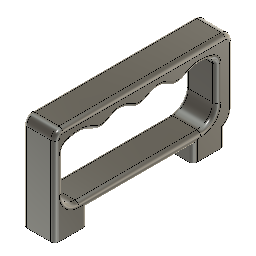
main (Autodesk Fusion 360 archive; units mm, degrees)
design "main_handle"
Autodesk Fusion 360 part; units mm, degrees
sketch "Skizze1" plane through (0, 0, 0) normal (1, 0, 0) x (0, 1, 0)
  line L0 (0, 0) -> (0, 60)
  line L1 (0, 60) -> (111.25, 60)
  line L2 (111.25, 60) -> (111.25, 10)
  line L3 (111.25, 10) -> (106.25, 10)
  line L4 (106.25, 10) -> (106.25, 0)
  line L5 (106.25, 0) -> (86.25, 0)
  line L6 (86.25, 0) -> (86.25, 10)
  line L7 (86.25, 10) -> (20, 10)
  line L8 (20, 10) -> (20, 0)
  line L9 (20, 0) -> (0, 0)
  dimension "d1" = 20
  dimension "d2" = 20
  dimension "d3" = 86.25
  dimension "d4" = 5
  dimension "d5" = 60
  dimension "d6" = 10
  dimension "d7" = 10
  constraint coincident L0.start L9.end
  constraint vertical L0
  constraint perpendicular L0 L1
  constraint perpendicular L1 L2
  constraint perpendicular L2 L3
  constraint perpendicular L3 L4
  constraint perpendicular L4 L5
  constraint perpendicular L3 L6
  constraint perpendicular L6 L7
  constraint perpendicular L3 L8
  constraint perpendicular L0 L9
  constraint collinear L5 L9
  measures "d1" distance of L8.end L0.start
  measures "d2" distance of L4.end L5.end
  measures "d3" distance of L0 L6
  measures "d4" distance of L2.end L3.end
  measures "d5" distance of L0.start L0.end
  measures "d6" distance of L7.end L8.end
  measures "d7" distance of L3.end L4.end
extrude "Extrusion1" add sketch "Skizze1" along normal mid plane 20
sketch "Skizze2" plane through (10, 0, 0) normal (1, 0, 0) x (0, 1, 0)
  line L0 (20, 0) -> (20, 10)
  line L1 (20, 10) -> (86.25, 10)
  line L2 (86.25, 10) -> (86.25, 0)
  line L3 (86.25, 0) -> (106.25, 0)
  line L4 (106.25, 0) -> (106.25, 10)
  line L5 (106.25, 10) -> (111.25, 10)
  line L6 (111.25, 10) -> (111.25, 60)
  line L7 (111.25, 60) -> (0, 60)
  line L8 (0, 60) -> (0, 0)
  line L9 (0, 0) -> (20, 0)
  spline S0 degree 5 poles (5, 50) (5.4629, 50.1553) (6.3735, 50.4513) (7.694, 50.8519) (9.3638, 51.2991) (11.3005, 51.7132) (13.0897, 51.9831) (14.7376, 52.1102) (16.2549, 52.0972) (17.6578, 51.9482) (18.9696, 51.669) (20.2192, 51.2688) (21.4368, 50.7637) (22.6495, 50.1803) (23.8773, 49.5586) (25.128, 48.9571) (26.3991, 48.445) (27.6823, 48.0889) (28.9673, 47.9419) (30.2456, 48.0313) (31.5144, 48.3467) (32.7751, 48.8486) (34.0317, 49.4766) (35.2885, 50.1586) (36.5487, 50.8196) (37.8129, 51.3893) (39.0803, 51.8072) (40.349, 52.0283) (41.6173, 52.0271) (42.8839, 51.8047) (44.1488, 51.3883) (45.4125, 50.8244) (46.6756, 50.1733) (47.9391, 49.5031) (49.2032, 48.8845) (50.4682, 48.3839) (51.7339, 48.0572) (53, 47.9433) (54.2661, 48.0572) (55.5318, 48.3839) (56.7968, 48.8845) (58.0609, 49.5031) (59.3244, 50.1733) (60.5875, 50.8244) (61.8512, 51.3883) (63.1161, 51.8047) (64.3827, 52.0271) (65.651, 52.0283) (66.9197, 51.8072) (68.1871, 51.3893) (69.4513, 50.8196) (70.7115, 50.1586) (71.9683, 49.4766) (73.2249, 48.8486) (74.4856, 48.3467) (75.7544, 48.0313) (77.0327, 47.9419) (78.3177, 48.0889) (79.6009, 48.445) (80.872, 48.9571) (82.1227, 49.5586) (83.3505, 50.1803) (84.5632, 50.7637) (85.7808, 51.2688) (87.0304, 51.669) (88.3422, 51.9482) (89.7451, 52.0972) (91.2624, 52.1102) (92.9103, 51.9831) (94.6995, 51.7132) (96.6362, 51.2991) (98.306, 50.8519) (99.6265, 50.4513) (100.5371, 50.1553) (101, 50) knots 0 0 0 0 0 0 0.01428571 0.02857143 0.04285714 0.05714286 0.07142857 0.08571429 0.1 0.11428571 0.12857143 0.14285714 0.15714286 0.17142857 0.18571429 0.2 0.21428571 0.22857143 0.24285714 0.25714286 0.27142857 0.28571429 0.3 0.31428571 0.32857143 0.34285714 0.35714286 0.37142857 0.38571429 0.4 0.41428571 0.42857143 0.44285714 0.45714286 0.47142857 0.48571429 0.5 0.51428571 0.52857143 0.54285714 0.55714286 0.57142857 0.58571429 0.6 0.61428571 0.62857143 0.64285714 0.65714286 0.67142857 0.68571429 0.7 0.71428571 0.72857143 0.74285714 0.75714286 0.77142857 0.78571429 0.8 0.81428571 0.82857143 0.84285714 0.85714286 0.87142857 0.88571429 0.9 0.91428571 0.92857143 0.94285714 0.95714286 0.97142857 0.98571429 1 1 1 1 1 1
  line L10 (5, 50) -> (101, 50)
  line L11 (5, 50) -> (5, 15)
  line L12 (5, 15) -> (101, 15)
  line L13 (101, 15) -> (101, 50)
  point P0 (17, 52)
  point P1 (23, 50)
  point P2 (29, 48)
  point P3 (35, 50)
  point P4 (41, 52)
  point P5 (47, 50)
  point P6 (53, 48)
  point P7 (59, 50)
  point P8 (65, 52)
  point P9 (71, 50)
  point P10 (77, 48)
  point P11 (83, 50)
  point P12 (89, 52)
  dimension "d10" = 5
  dimension "d11" = 12
  dimension "d12" = 6
  dimension "d13" = 6
  dimension "d14" = 6
  dimension "d15" = 6
  dimension "d16" = 6
  dimension "d17" = 6
  dimension "d18" = 6
  dimension "d19" = 6
  dimension "d20" = 6
  dimension "d21" = 6
  dimension "d22" = 6
  dimension "d24" = 10
  dimension "d25" = 10
  dimension "d26" = 6
  dimension "d27" = 12
  dimension "d28" = 2
  dimension "d29" = 2
  dimension "d30" = 2
  dimension "d31" = 2
  dimension "d32" = 2
  dimension "d33" = 2
  dimension "d34" = 2
  dimension "d35" = 35
  constraint coincident P1 L10
  constraint coincident P3 L10
  constraint coincident P5 L10
  constraint coincident P7 L10
  constraint coincident P9 L10
  constraint coincident P11 L10
  constraint perpendicular L10 L11
  constraint perpendicular L11 L12
  constraint perpendicular L10 L13
  measures "d10" distance of L8 S0.start
  measures "d11" distance of S0.start P0
  measures "d12" horizontal distance of P0 P1
  measures "d13" horizontal distance of P1 P2
  measures "d14" horizontal distance of P2 P3
  measures "d15" horizontal distance of P3 P4
  measures "d16" horizontal distance of P4 P5
  measures "d17" horizontal distance of P5 P6
  measures "d18" horizontal distance of P6 P7
  measures "d19" horizontal distance of P7 P8
  measures "d20" horizontal distance of P8 P9
  measures "d21" horizontal distance of P9 P10
  measures "d22" horizontal distance of P10 P11
  measures "d24" distance of L7 S0.end
  measures "d25" distance of L7 S0.start
  measures "d26" horizontal distance of P11 P12
  measures "d27" distance of S0.end P12
  measures "d28" distance of L10 P12
  measures "d29" distance of P10 L10
  measures "d30" distance of P8 L10
  measures "d31" distance of P6 L10
  measures "d32" distance of P4 L10
  measures "d33" distance of P2 L10
  measures "d34" distance of P0 L10
  measures "d35" distance of S0.start L11.end
extrude "Extrusion2" cut sketch "Skizze2" against normal through all contours S0 L10 | S0 L10 L11 L12 L13 | S0 L10 | S0 L10 | S0 L10 picked at (13.1167, 50.5643) picked at (39.3753, 50.6892) picked at (93.7853, 50.364) picked at (66.4503, 50.2815)
fillet "Abrundung11" radius 10 3 edges at (0, 101, 15) (0, 111.25, 10) (0, 5, 15)
fillet "Abrundung12" radius 5 2 edges at (0, 111.25, 60) (0, 0, 60)
fillet "Abrundung13" radius 5 2 edges at (0, 101, 50) (0, 5, 50)
fillet "Abrundung14" radius 2.5 28 edges at (-10, 0, 27.5) (-10, 1.4645, 58.5355) (-10, 55.625, 60) (-10, 109.7855, 58.5355) (-10, 111.25, 36.8301) (-10, 109.9103, 13.6603) (-10, 6.0478, 49.3407) (-10, 53, 48) (-10, 99.9489, 49.3449) (-10, 101, 35.639) (-10, 98.0711, 17.9289) (-10, 53, 15) (-10, 7.9289, 17.9289) (-10, 5, 35.639) (10, 7.9289, 17.9289) (10, 53, 15) (10, 98.0711, 17.9289) (10, 101, 35.639) (10, 99.9522, 49.3407) (10, 53, 48) (10, 6.0511, 49.3449) (10, 5, 35.639) (10, 109.9103, 13.6603) (10, 111.25, 36.8301) (10, 109.7855, 58.5355) (10, 55.625, 60) (10, 1.4645, 58.5355) (10, 0, 27.5)
fillet "Abrundung15" radius 2.5 2 edges at (-10, 53.125, 10) (10, 53.125, 10)
fillet "Abrundung16" radius 2.5 6 edges at (-10, 86.25, 6.25) (10, 86.25, 6.25) (10, 106.25, 6.535) (-10, 106.25, 6.535) (-10, 20, 6.25) (10, 20, 6.25)
sketch "Skizze3" plane through (0, 0, 0) normal (0, 0, -1) x (1, 0, 0)
  arc A0 (-10, -103.75) -> (-7.5, -106.25) centre (-7.5, -103.75) ccw
  line L0 (-7.5, -106.25) -> (7.5, -106.25)
  arc A1 (7.5, -106.25) -> (10, -103.75) centre (7.5, -103.75) ccw
  line L1 (10, -103.75) -> (10, -88.75)
  arc A2 (10, -88.75) -> (7.5, -86.25) centre (7.5, -88.75) ccw
  line L2 (7.5, -86.25) -> (-7.5, -86.25)
  arc A3 (-7.5, -86.25) -> (-10, -88.75) centre (-7.5, -88.75) ccw
  line L3 (-10, -88.75) -> (-10, -103.75)
  line L4 (0, -1.75) -> (0, -22.5)
  point P0 (0, -96.25)
  point P1 (0, -10)
  dimension "d69" = 86.25
  dimension "d70" = 10
  constraint coincident P1 L4
  constraint coincident P0 L4
  measures "d69" distance of P0 P1
  measures "d70" distance of L0 P0
hole "Bohrung1" at (0, 96.25, 0) at (0, 10, 0) direction (0, 0, 1) diameter 3.2 depth 14 tip angle 180
ref_plane "Arbeitsebene2" through (0, 96.25, 5) normal (0, 0, -1) x (0, 1, 0)
sketch "Skizze12" plane through (0, 96.25, 5) normal (0, 0, -1) x (1, 0, 0)
  line L0 (2.9, 89.85) -> (-2.9, 89.85)
  line L1 (-2.9, 89.85) -> (-2.9, -3.6)
  line L2 (-2.9, -3.6) -> (2.9, -3.6)
  line L3 (2.9, -3.6) -> (2.9, 89.85)
  point P0 (-1.6, 86.25)
  dimension "d119" = 5.8
  dimension "d120" = 3.6
  dimension "d121" = 2.9
  dimension "d122" = 3.6
  constraint horizontal L0
  constraint vertical L1
  constraint horizontal L2
  constraint vertical L3
  measures "d119" distance of L1.end L2.end
  measures "d120" distance of origin L2
  measures "d121" distance of origin L3
  measures "d122" vertical distance of L0.end P0
extrude "Extrusion10" cut sketch "Skizze12" against normal blind 3
sketch "Skizze13" plane through (0, 0, 0) normal (1, 0, 0) x (0, 1, 0)
  line L0 (111.25, 18.6603) -> (111.25, 55)
  line L1 (88.75, 0) -> (103.75, 0)
  line L2 (111.25, 50) -> (106.75, 50)
  line L3 (106.75, 50) -> (106.75, 45)
  line L4 (106.75, 45) -> (104.75, 45)
  line L5 (104.75, 45) -> (104.75, 19.017)
  line L6 (104.75, 19.017) -> (102.25, 15.4466)
  line L7 (102.25, 15.4466) -> (102.25, 0)
  line L8 (105.25, 0) -> (105.25, 14.5007)
  line L9 (105.25, 14.5007) -> (107, 17)
  line L10 (107, 17) -> (107, 42.5)
  line L11 (107, 42.5) -> (108.25, 42.5)
  line L12 (108.25, 42.5) -> (108.25, 43.5)
  line L13 (108.25, 43.5) -> (111.25, 43.5)
  line L14 (111.25, 43.5) -> (111.25, 50)
  line L15 (106.25, 60) -> (5, 60)
  line L16 (102.25, 0) -> (105.25, 0)
  dimension "d128" = 4.5
  dimension "d129" = 2
  dimension "d130" = 3
  dimension "d131" = 2.25
  dimension "d132" = 2.5
  dimension "d133" = 5
  dimension "d134" = 6.5
  dimension "d135" = 10
  dimension "d137" = 145
  dimension "d138" = 2.5
  dimension "d139" = 3
  dimension "d140" = 3
  dimension "d141" = 28
  constraint coincident L0 L2.start
  constraint perpendicular L0 L2
  constraint perpendicular L2 L3
  constraint perpendicular L3 L4
  constraint perpendicular L4 L5
  constraint coincident L1 L7.end
  constraint perpendicular L1 L7
  constraint coincident L1 L8.start
  constraint perpendicular L1 L8
  constraint parallel L6 L9
  constraint perpendicular L1 L10
  constraint perpendicular L7 L11
  constraint perpendicular L11 L12
  constraint coincident L0 L13.end
  constraint perpendicular L0 L13
  measures "d128" distance of L2.start L2.end
  measures "d129" distance of L3.end L4.end
  measures "d130" distance of L12.end L13.end
  measures "d131" distance of L5 L10
  measures "d132" distance of L4 L11
  measures "d133" distance of L2.end L3.end
  measures "d134" distance of L2.start L13.end
  measures "d135" distance of L2 L15
  measures "d137" angle of L5 L6
  measures "d138" horizontal distance of L5.end L6.end
  measures "d139" distance of L7 L8
  measures "d140" distance of L6 L9
  measures "d141" vertical distance of L4.end L9.end
extrude "Extrusion11" cut sketch "Skizze13" along normal mid plane 6.5
equation "d11 = fingerdist * 2"
equation "d12 = fingerdist"
equation "d13 = fingerdist"
equation "d14 = fingerdist"
equation "d15 = fingerdist"
equation "d16 = fingerdist"
equation "d17 = fingerdist"
equation "d18 = fingerdist"
equation "d19 = fingerdist"
equation "d20 = fingerdist"
equation "d21 = fingerdist"
equation "d22 = fingerdist"
equation "d26 = fingerdist"
equation "d27 = fingerdist * 2"
equation "fingerdist = 6 mm"

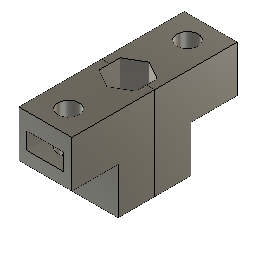
design "module_stand"
Autodesk Fusion 360 part; units mm, degrees
sketch "Skizze1" plane through (0, 0, 0) normal (1, 0, 0) x (0, 1, 0)
  line L0 (0, 0) -> (0, 14)
  line L1 (0, 14) -> (12.5, 14)
  line L2 (12.5, 14) -> (12.5, 7)
  line L3 (12.5, 7) -> (5.5, 7)
  line L4 (5.5, 7) -> (5.5, 0)
  line L5 (5.5, 0) -> (0, 0)
  dimension "d1" = 5.5
  dimension "d2" = 7
  dimension "d3" = 14
  dimension "d4" = 12.5
  constraint coincident L0.start L5.end
  constraint vertical L0
  constraint perpendicular L0 L1
  constraint perpendicular L1 L2
  constraint perpendicular L2 L3
  constraint perpendicular L1 L4
  constraint perpendicular L4 L5
  measures "d1" distance of L0.start L4.end
  measures "d2" distance of L3.end L4.end
  measures "d3" distance of L0.start L0.end
  measures "d4" distance of L0.end L1.end
extrude "Extrusion1" add sketch "Skizze1" along normal blind 8 makes body 1
sketch "Skizze2" plane through (0, 0, 14) normal (0, 0, 1) x (-1, 0, 0)
  line L0 (0, -12.5) -> (0, 0)
  line L1 (0, 0) -> (-8, 0)
  line L2 (-8, 0) -> (-8, -12.5)
  line L3 (-8, -12.5) -> (0, -12.5)
  point P0 (-4, 0)
  point P1 (-4, -9)
  dimension "d7" = 4
  dimension "d8" = 4
  dimension "d10" = 3.5
  constraint coincident L1 P0
  measures "d7" distance of L2 P1
  measures "d8" distance of L2 P0
  measures "d10" distance of L3 P1
hole "Bohrung1" at (4, 0, 14) at (4, 9, 14) direction (0, 0, -1) diameter 3.2 end through all bodies 1
sketch "Skizze3" plane through (0, 0, 14) normal (0, 0, 1) x (-1, 0, 0)
  arc A0 (-5.6, 0) -> (-2.4, 0) centre (-4, 0) ccw
  line L0 (-5.6, 0) -> (-8, 0)
  line L1 (-8, 0) -> (-8, -12.5)
  line L2 (-8, -12.5) -> (0, -12.5)
  line L3 (0, -12.5) -> (0, 0)
  line L4 (0, 0) -> (-2.4, 0)
  circle A1 centre (-4, -9) radius 1.6
  line L5 (-1.2, 1.6166) -> (-4, 3.2332)
  line L6 (-4, 3.2332) -> (-6.8, 1.6166)
  line L7 (-6.8, 1.6166) -> (-6.8, -1.6166)
  line L8 (-6.8, -1.6166) -> (-4, -3.2332)
  line L9 (-4, -3.2332) -> (-1.2, -1.6166)
  line L10 (-1.2, -1.6166) -> (-1.2, 1.6166)
  point P0 (-4, 0)
  dimension "d14" = 5.6
  constraint coincident P0 A0.centre
  constraint parallel L1 L7
  measures "d14" distance of L7 L10
extrude "Extrusion2" cut sketch "Skizze3" against normal blind 7 contours A0 L0 L4 L7 L8 L9 L10 bodies 1
sketch "Skizze5" plane through (0, 12.5, 0) normal (0, 1, 0) x (-1, 0, 0)
  line L0 (0, 7) -> (0, 14)
  line L1 (0, 14) -> (-8, 14)
  line L2 (-8, 14) -> (-8, 7)
  line L3 (-8, 7) -> (0, 7)
  line L4 (-6.8, 11.5) -> (-1.2, 11.5)
  line L5 (-1.2, 11.5) -> (-1.2, 8.9)
  line L6 (-1.2, 8.9) -> (-6.8, 8.9)
  line L7 (-6.8, 8.9) -> (-6.8, 11.5)
  dimension "d22" = 5.6
  dimension "d23" = 2.6
  dimension "d24" = 2.5
  dimension "d25" = 1.2
  dimension "d26" = 8
  constraint horizontal L4
  constraint vertical L5
  constraint horizontal L6
  constraint vertical L7
  measures "d22" distance of L5.end L6.end
  measures "d23" distance of L4.end L5.end
  measures "d24" distance of L1 L4
  measures "d25" distance of L0 L5
  measures "d26" distance of L0.end L1.end
extrude "Extrusion4" cut sketch "Skizze5" against normal blind 6.7 contours L4 L5 L6 L7 bodies 1
mirror "Spiegeln1" about plane through (0, 0, 0) normal (0, -1, 0) of "Extrusion1", "Bohrung1", "Extrusion2", "Extrusion4" makes body 2
equation "d1 = ( 11 / 2 ) * 1 mm"
equation "d4 = ( 25 / 2 ) * 1 mm"
equation "d25 = ( 8.00 mm - d22 ) / 2"

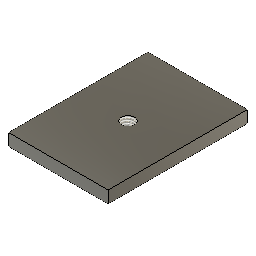
design "module_plate"
Autodesk Fusion 360 part; units mm, degrees
sketch "Skizze1" plane through (0, 0, 0) normal (0, 0, 1) x (1, 0, 0)
  line L0 (-12.5, -17.5) -> (12.5, -17.5)
  line L1 (12.5, -17.5) -> (12.5, 17.5)
  line L2 (12.5, 17.5) -> (-12.5, 17.5)
  line L3 (-12.5, 17.5) -> (-12.5, -17.5)
  dimension "d1" = 25
  dimension "d2" = 35
  dimension "d3" = 17.5
  dimension "d4" = 12.5
  constraint horizontal L0
  constraint vertical L1
  constraint horizontal L2
  constraint vertical L3
  measures "d1" distance of L0.start L0.end
  measures "d2" distance of L0.end L1.end
  measures "d3" distance of origin L2
  measures "d4" distance of origin L3
extrude "Extrusion1" add sketch "Skizze1" along normal blind 3
sketch "Skizze2" plane through (0, 0, 3) normal (0, 0, 1) x (-1, 0, 0)
  line L0 (12.5, -17.5) -> (12.5, 17.5)
  line L1 (12.5, 17.5) -> (-12.5, 17.5)
  line L2 (-12.5, 17.5) -> (-12.5, -17.5)
  line L3 (-12.5, -17.5) -> (12.5, -17.5)
hole "Bohrung1" at (0, 0, 3) direction (0, 0, -1) diameter 3.332 end through all
thread "Gewinde1" "ISO Metric profile 4.0 M4x0.7 6H"
equation "d3 = ( 35 / 2 ) * 1 mm"
equation "d4 = ( 25 / 2 ) * 1 mm"

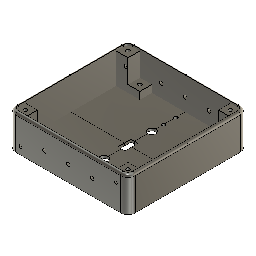
design "main_case"
Autodesk Fusion 360 part; units mm, degrees
sketch "Skizze1" plane through (0, 0, 0) normal (0, 0, 1) x (1, 0, 0)
  line L0 (0, 0) -> (50, 0)
  line L1 (50, 0) -> (50, 50)
  line L2 (50, 50) -> (0, 50)
  line L3 (0, 50) -> (0, 0)
  dimension "d1" = 50
  dimension "d2" = 50
  constraint horizontal L0
  constraint vertical L1
  constraint horizontal L2
  constraint vertical L3
  constraint coincident L0.start L3.end
  measures "d1" distance of L0.start L0.end
  measures "d2" distance of L0.end L1.end
extrude "Extrusion1" add sketch "Skizze1" along normal blind 29 makes body 1
sketch "Skizze2" plane through (0, 0, 29) normal (0, 0, 1) x (-1, 0, 0)
  line L0 (0, -50) -> (0, 0)
  line L1 (0, 0) -> (-50, 0)
  line L2 (-50, 0) -> (-50, -50)
  line L3 (-50, -50) -> (0, -50)
  line L4 (0, 0) -> (-48, 0)
  line L5 (-48, 0) -> (-48, -48)
  line L6 (-48, -48) -> (0, -48)
  line L7 (0, -48) -> (0, 0)
  dimension "d5" = 2
  dimension "d6" = 2
  constraint horizontal L4
  constraint vertical L5
  constraint horizontal L6
  constraint vertical L7
  constraint coincident L0.end L1.start
  measures "d5" distance of L2 L5
  measures "d6" distance of L3 L6
extrude "Extrusion2" cut sketch "Skizze2" against normal blind 27 contours L0 L1 L4 L5 L6 L7 bodies 1
sketch "Skizze3" plane through (0, 0, 2) normal (0, 0, 1) x (-1, 0, 0)
  line L0 (0, -48) -> (0, 0)
  line L1 (0, 0) -> (-48, 0)
  line L2 (-48, 0) -> (-48, -48)
  line L3 (-48, -48) -> (0, -48)
  line L4 (-48, -48) -> (-38, -48)
  line L5 (-38, -48) -> (-38, -38)
  line L6 (-38, -38) -> (-48, -38)
  line L7 (-48, -38) -> (-48, -48)
  dimension "d9" = 10
  dimension "d10" = 10
  constraint horizontal L4
  constraint vertical L5
  constraint horizontal L6
  constraint vertical L7
  constraint coincident L2.end L3.start
  measures "d9" distance of L5.end L6.end
  measures "d10" distance of L4.end L5.end
extrude "Extrusion3" add sketch "Skizze3" along normal blind 25.4 contours L2 L3 L4 L5 L6 L7 bodies 1
sketch "Skizze4" plane through (0, 0, 2) normal (0, 0, 1) x (-1, 0, 0)
  line L0 (-48, -38) -> (-38, -38)
  line L1 (-38, -38) -> (-38, -48)
  line L2 (-38, -48) -> (0, -48)
  line L3 (0, -48) -> (0, 0)
  line L4 (0, 0) -> (-48, 0)
  line L5 (-48, 0) -> (-48, -38)
  line L6 (0, 0) -> (-3.04, 0)
  line L7 (-3.04, 0) -> (-3.04, -5.58)
  line L8 (-3.04, -5.58) -> (0, -5.58)
  line L9 (0, -5.58) -> (0, 0)
  dimension "d13" = 3.04
  dimension "d14" = 5.58
  constraint horizontal L6
  constraint vertical L7
  constraint horizontal L8
  constraint vertical L9
  constraint coincident L3.end L4.start
  measures "d13" distance of L3.end L6.end
  measures "d14" distance of L6.end L7.end
extrude "Extrusion4" cut sketch "Skizze4" against normal through all contours L3 L4 L6 L7 L8 L9 bodies 1
sketch "Skizze5" plane through (0, 0, 2) normal (0, 0, 1) x (-1, 0, 0)
  line L0 (0, -5.58) -> (-3.04, -5.58)
  line L1 (-3.04, -5.58) -> (-3.04, 0)
  line L2 (-3.04, 0) -> (-48, 0)
  line L3 (-48, 0) -> (-48, -38)
  line L4 (-48, -38) -> (-38, -38)
  line L5 (-38, -38) -> (-38, -48)
  line L6 (-38, -48) -> (0, -48)
  line L7 (0, -48) -> (0, -5.58)
  point P0 (0, -40)
  dimension "d17" = 40
  constraint coincident L7 P0
  measures "d17" distance of L2 P0
hole "Bohrung1" at (0, 40, 2) direction (0, 0, -1) diameter 3.2 depth 10 tip angle 118 bodies 1
sketch "Skizze6" plane through (0, 0, 27.4) normal (0, 0, 1) x (-1, 0, 0)
  line L0 (-38, -48) -> (-38, -38)
  line L1 (-38, -38) -> (-48, -38)
  line L2 (-48, -38) -> (-48, -48)
  line L3 (-48, -48) -> (-38, -48)
  point P0 (-43, -43)
hole "Bohrung2" at (43, 43, 27.4) direction (0, 0, -1) diameter 3.2 end through all bodies 1
sketch "Skizze7" plane through (0, 0, 0) normal (0, 0, -1) x (1, 0, 0)
  line L0 (0, -41.6) -> (0, -50)
  line L1 (0, -50) -> (50, -50)
  line L2 (50, -50) -> (50, 0)
  line L3 (50, 0) -> (3.04, 0)
  line L4 (41.3257, -40.1) -> (39.6514, -43)
  line L5 (39.6514, -43) -> (41.3257, -45.9)
  line L6 (41.3257, -45.9) -> (44.6743, -45.9)
  line L7 (44.6743, -45.9) -> (46.3486, -43)
  line L8 (46.3486, -43) -> (44.6743, -40.1)
  line L9 (44.6743, -40.1) -> (41.3257, -40.1)
  circle A0 centre (43, -43) radius 1.6
  arc A1 (0, -41.6) -> (0, -38.4) centre (0, -40) ccw
  line L10 (3.04, 0) -> (3.04, -5.58)
  line L11 (3.04, -5.58) -> (0, -5.58)
  line L12 (0, -5.58) -> (0, -38.4)
  point P0 (43, -43)
  dimension "d26" = 5.8
  constraint parallel L1 L6
  constraint coincident P0 A0.centre
  measures "d26" distance of L6 L9
extrude "Extrusion5" cut sketch "Skizze7" against normal blind 12.5 contours L4 L5 L6 L7 L8 L9 | A0 bodies 1
fillet "Abrundung1" radius 4 1 edges at (48, 48, 28.2) on bodies 1
fillet "Abrundung2" radius 6 1 edges at (50, 50, 14.5) on bodies 1
sketch "Skizze8" plane through (0, 0, 2) normal (0, 0, 1) x (-1, 0, 0)
  arc A0 (0, -38.4) -> (0, -41.6) centre (0, -40) ccw
  line L0 (0, -38.4) -> (0, -5.58)
  line L1 (0, -5.58) -> (-3.04, -5.58)
  line L2 (-3.04, -5.58) -> (-3.04, 0)
  line L3 (-3.04, 0) -> (-48, 0)
  line L4 (-48, 0) -> (-48, -38)
  line L5 (-48, -38) -> (-38, -38)
  line L6 (-38, -38) -> (-38, -48)
  line L7 (-38, -48) -> (0, -48)
  line L8 (0, -48) -> (0, -41.6)
  line L9 (-38, -38) -> (-28, -38)
  line L10 (-28, -38) -> (-28, -48)
  line L11 (-28, -48) -> (-38, -48)
  line L12 (-38, -48) -> (-38, -38)
  dimension "d35" = 10
  dimension "d36" = 10
  constraint horizontal L9
  constraint vertical L10
  constraint horizontal L11
  constraint vertical L12
  constraint coincident L7 L10.end
  constraint coincident L6 L5.end
  measures "d35" distance of L5.end L9.end
  measures "d36" distance of L9.end L10.end
extrude "Extrusion6" add sketch "Skizze8" along normal blind 6 contours L6 L7 L9 L10 L11 L12 bodies 1
sketch "Skizze9" plane through (0, 0, 8) normal (0, 0, 1) x (-1, 0, 0)
  line L0 (-38, -48) -> (-28, -48)
  line L1 (-28, -48) -> (-28, -38)
  line L2 (-28, -38) -> (-38, -38)
  line L3 (-38, -38) -> (-38, -48)
  point P0 (-33, -43)
  dimension "d39" = 5
  dimension "d40" = 5
  measures "d39" distance of L0 P0
  measures "d40" distance of L3 P0
hole "Bohrung3" at (33, 43, 8) direction (0, 0, -1) diameter 3.2 end through all bodies 1
sketch "Skizze10" plane through (0, 0, 0) normal (0, 0, -1) x (1, 0, 0)
  arc A0 (44, -50) -> (50, -44) centre (44, -44) ccw
  line L0 (50, -44) -> (50, 0)
  line L1 (50, 0) -> (3.04, 0)
  line L2 (0, -5.58) -> (0, -38.4)
  line L3 (0, -50) -> (44, -50)
  line L4 (31.3257, -40.1) -> (29.6514, -43)
  line L5 (29.6514, -43) -> (31.3257, -45.9)
  line L6 (31.3257, -45.9) -> (34.6743, -45.9)
  line L7 (34.6743, -45.9) -> (36.3486, -43)
  line L8 (36.3486, -43) -> (34.6743, -40.1)
  line L9 (34.6743, -40.1) -> (31.3257, -40.1)
  circle A1 centre (33, -43) radius 1.6
  line L10 (44.6743, -45.9) -> (41.3257, -45.9)
  line L11 (41.3257, -45.9) -> (39.6514, -43)
  line L12 (39.6514, -43) -> (41.3257, -40.1)
  line L13 (41.3257, -40.1) -> (44.6743, -40.1)
  line L14 (44.6743, -40.1) -> (46.3486, -43)
  line L15 (46.3486, -43) -> (44.6743, -45.9)
  line L16 (3.04, 0) -> (3.04, -5.58)
  line L17 (3.04, -5.58) -> (0, -5.58)
  arc A2 (0, -41.6) -> (0, -38.4) centre (0, -40) ccw
  line L18 (0, -41.6) -> (0, -50)
  point P0 (33, -43)
  dimension "d44" = 5.8
  constraint parallel L3 L6
  measures "d44" distance of L6 L9
extrude "Extrusion7" cut sketch "Skizze10" against normal blind 4 contours L4 L5 L6 L7 L8 L9 | A1 bodies 1
fillet "Abrundung4" radius 2 3 edges at (50, 22, 29) (48.2426, 48.2426, 29) (22, 50, 29) on bodies 1
sketch "Skizze14" plane through (0, 0, 2) normal (0, 0, 1) x (-1, 0, 0)
  line L0 (-28, -38) -> (-28, -48)
  line L1 (-28, -48) -> (0, -48)
  line L2 (0, -48) -> (0, -41.6)
  arc A0 (0, -38.4) -> (0, -41.6) centre (0, -40) ccw
  line L3 (0, -38.4) -> (0, -5.58)
  line L4 (0, -5.58) -> (-3.04, -5.58)
  line L5 (-3.04, -5.58) -> (-3.04, 0)
  line L6 (-3.04, 0) -> (-48, 0)
  line L7 (-48, 0) -> (-48, -38)
  line L8 (-48, -38) -> (-28, -38)
  point P0 (0, -20)
  dimension "d79" = 20
  constraint coincident L3 P0
  measures "d79" distance of L6 P0
hole "Bohrung7" at (0, 20, 2) direction (0, 0, -1) diameter 7 end through all bodies 1
mirror "Spiegeln1" about plane through (0, 0, 0) normal (1, 0, 0) of "Extrusion1", "Extrusion2", "Extrusion3", "Extrusion4", "Bohrung1", "Bohrung2", "Extrusion5", "Abrundung1", "Abrundung2", "Extrusion6", "Bohrung3", "Extrusion7", "Abrundung4", "Bohrung7" makes body 2
mirror "Spiegeln2" about plane through (0, 0, 0) normal (0, 1, 0) of "Extrusion1", "Extrusion2", "Extrusion3", "Extrusion4", "Bohrung1", "Bohrung2", "Extrusion5", "Abrundung1", "Abrundung2", "Extrusion6", "Bohrung3", "Extrusion7", "Abrundung4", "Bohrung7", "Spiegeln1" makes body 3 at (28.246, -19.7737, 0) makes body 4 at (-28.246, -19.7737, 0)
sketch "Skizze11" plane through (0, -50, 0) normal (0, -1, 0) x (1, 0, 0)
  line L0 (0, 27) -> (-44, 27)
  line L1 (-44, 27) -> (-44, 0)
  line L2 (-44, 0) -> (0, 0)
  line L3 (0, 0) -> (0, 27)
  line L4 (44, 0) -> (0, 0)
  point P0 (0, 13)
  point P1 (20, 13)
  point P2 (-20, 13)
  dimension "d56" = 20
  dimension "d57" = 20
  dimension "d58" = 13
  dimension "d59" = 27
  dimension "d60" = 13
  dimension "d61" = 13
  constraint coincident L3 P0
  measures "d56" distance of P0 P1
  measures "d57" distance of P0 P2
  measures "d58" distance of L2 P2
  measures "d59" distance of L0 L2
  measures "d60" distance of P0 L4
  measures "d61" distance of P1 L4
hole "Bohrung4" at (20, -50, 13) at (0, -50, 13) at (-20, -50, 13) direction (0, 1, 0) diameter 3.2 end through all bodies 1 2 3 4
sketch "Skizze12" plane through (0, -50, 0) normal (0, -1, 0) x (1, 0, 0)
  arc A0 (0, 14.6) -> (0, 11.4) centre (0, 13) ccw
  line L0 (0, 14.6) -> (0, 27)
  line L1 (0, 27) -> (-44, 27)
  line L2 (-44, 27) -> (-44, 0)
  line L3 (-44, 0) -> (0, 0)
  line L4 (0, 0) -> (0, 11.4)
  circle A1 centre (-20, 13) radius 1.6
  circle A2 centre (20, 13) radius 1.6
  point P0 (40, 20)
  point P1 (-40, 6)
  dimension "d65" = 40
  dimension "d66" = 40
  dimension "d67" = 7
  dimension "d68" = 7
  measures "d65" horizontal distance of A0.centre P1
  measures "d66" horizontal distance of A0.centre P0
  measures "d67" vertical distance of P0 A2.centre
  measures "d68" vertical distance of A1.centre P1
hole "Bohrung5" at (-40, -50, 6) at (40, -50, 20) direction (0, 1, 0) diameter 2.5 depth 20 tip angle 118 bodies 3 4
sketch "Skizze13" plane through (0, 50, 0) normal (0, 1, 0) x (-1, 0, 0)
  arc A0 (0, 11.4) -> (0, 14.6) centre (0, 13) ccw
  line L0 (0, 11.4) -> (0, 0)
  line L1 (0, 0) -> (44, 0)
  line L2 (44, 0) -> (44, 27)
  line L3 (44, 27) -> (0, 27)
  line L4 (0, 27) -> (0, 14.6)
  circle A1 centre (20, 13) radius 1.6
  circle A2 centre (-20, 13) radius 1.6
  point P0 (40, 20)
  point P1 (-40, 6)
  dimension "d72" = 40
  dimension "d73" = 7
  dimension "d74" = 40
  dimension "d75" = 7
  measures "d72" horizontal distance of A0.centre P1
  measures "d73" vertical distance of P1 A2.centre
  measures "d74" horizontal distance of A0.centre P0
  measures "d75" vertical distance of A1.centre P0
hole "Bohrung6" at (-40, 50, 20) at (40, 50, 6) direction (0, -1, 0) diameter 2.5 depth 20 tip angle 118 bodies 1 2
sketch "Skizze15" plane through (0, 0, 2) normal (0, 0, 1) x (-1, 0, 0)
  arc A0 (0, -16.5) -> (0, -23.5) centre (0, -20) ccw
  line L0 (0, -16.5) -> (0, -5.58)
  line L1 (0, -5.58) -> (-3.04, -5.58)
  line L2 (-3.04, -5.58) -> (-3.04, 0)
  line L3 (-3.04, 0) -> (-48, 0)
  line L4 (-48, 0) -> (-48, -38)
  line L5 (-48, -38) -> (-28, -38)
  line L6 (-28, -38) -> (-28, -48)
  line L7 (-28, -48) -> (0, -48)
  line L8 (0, -48) -> (0, -41.6)
  arc A1 (0, -38.4) -> (0, -41.6) centre (0, -40) ccw
  line L9 (0, -38.4) -> (0, -23.5)
  point P0 (0, -30)
  dimension "d83" = 30
  constraint coincident L9 P0
  measures "d83" distance of origin P0
hole "Bohrung8" at (0, 30, 2) direction (0, 0, -1) diameter 3.2 end through all bodies 1 2
equation "d3 = height"
equation "d7 = -height + 2 mm"
equation "d11 = height - 2 mm - 1.6 mm"
equation "d13 = 2.54 mm + 0.5 mm"
equation "d14 = ( 2.54 * 2 ) * 1 mm + 0.5 mm"
equation "height = 29 mm"
equation "d58 = 26.00 mm / 2"

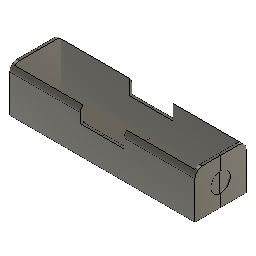
design "18620_holder"
Autodesk Fusion 360 part; units mm, degrees
sketch "Skizze1" plane through (0, 0, 0) normal (0, 0, 1) x (1, 0, 0)
  line L0 (0, 0) -> (38, 0)
  line L1 (38, 0) -> (38, 10.5)
  line L2 (38, 10.5) -> (0, 10.5)
  line L3 (0, 10.5) -> (0, 0)
  dimension "d1" = 38
  dimension "d2" = 10.5
  constraint horizontal L0
  constraint vertical L1
  constraint horizontal L2
  constraint vertical L3
  constraint coincident L0.start L3.end
  measures "d1" distance of L0.start L0.end
  measures "d2" distance of L0.end L1.end
extrude "Extrusion1" add sketch "Skizze1" along normal blind 18.5 makes body 1
shell "Schale1" thickness 1 removed faces 3 at (12.6667, 0, 6.1667) at (0, 3.5, 12.3333) at (25.3333, 3.5, 18.5) on bodies 1
fillet "Abrundung1" radius 3 1 edges at (19, 10.5, 18.5) on bodies 1
sketch "Skizze2" plane through (38, 0, 0) normal (1, 0, 0) x (0, 1, 0)
  arc A0 (10.5, 15.5) -> (7.5, 18.5) centre (7.5, 15.5) ccw
  line L0 (7.5, 18.5) -> (0, 18.5)
  line L1 (0, 18.5) -> (0, 0)
  line L2 (0, 0) -> (10.5, 0)
  line L3 (10.5, 0) -> (10.5, 15.5)
  circle A1 centre (0, 9) radius 4
  dimension "d8" = 9
  dimension "d9" = 8
  constraint coincident L1 A1.centre
  measures "d8" distance of L2 A1.centre
  measures "d9" diameter of A1
extrude "Extrusion2" cut sketch "Skizze2" against normal blind 0.5 contours L1 A1 picked at (1.594, 7.7807) bodies 1
sketch "Skizze3" plane through (0, 0, 18.5) normal (0, 0, 1) x (-1, 0, 0)
  line L0 (-38, -7.5) -> (-37, -7.5)
  line L1 (-37, -7.5) -> (-37, 0)
  line L2 (-37, 0) -> (-38, 0)
  line L3 (-38, 0) -> (-38, -7.5)
  line L4 (0, -9.5) -> (-9, -9.5)
  line L5 (-9, -9.5) -> (-9, -11.5)
  line L6 (-9, -11.5) -> (0, -11.5)
  line L7 (0, -11.5) -> (0, -9.5)
  line L8 (-37, 0) -> (0, 0)
  line L9 (0, 0) -> (0, -9.5)
  dimension "d12" = 9
  dimension "d13" = 2
  dimension "d14" = 9.5
  dimension "d16" = 29
  constraint horizontal L4
  constraint vertical L5
  constraint horizontal L6
  constraint vertical L7
  measures "d12" distance of L4.start L4.end
  measures "d13" distance of L4.end L5.end
  measures "d14" distance of L4 L8
  measures "d16" distance of L3 L5
extrude "Extrusion3" cut sketch "Skizze3" against normal blind 7 contours L4 L5 L6 L7 bodies 1
sketch "Skizze4" plane through (0, 0, 1) normal (0, 0, 1) x (-1, 0, 0)
  line L0 (0, -9.5) -> (0, 0)
  line L1 (0, 0) -> (-37, 0)
  line L2 (-37, 0) -> (-37, -9.5)
  line L3 (-37, -9.5) -> (0, -9.5)
  point P0 (-20, 0)
  dimension "d26" = 20
  constraint coincident L0.end L1.start
  constraint coincident L1 P0
  measures "d26" distance of L0.end P0
hole "Bohrung1" at (0, 0, 1) at (20, 0, 1) direction (0, 0, -1) diameter 3.2 depth 10 tip angle 118 bodies 1
mirror "Spiegeln1" about plane through (0, 0, 0) normal (0, 1, 0) of "Extrusion1", "Schale1", "Abrundung1", "Extrusion2", "Extrusion3", "Bohrung1" makes body 2
mirror "Spiegeln2" about plane through (0, 0, 0) normal (1, 0, 0) of "Extrusion1", "Schale1", "Abrundung1", "Extrusion2", "Extrusion3", "Bohrung1", "Spiegeln1" makes body 3 at (-27.6667, 9.5, 10.0787) makes body 4 at (-27.6667, -9.5, 10.0787)
equation "d1 = ( 76 / 2 ) * 1 mm"
equation "d2 = ( 21 / 2 ) * 1 mm"
equation "d16 = ( 76 / 2 ) * 1 mm - 9 mm"
